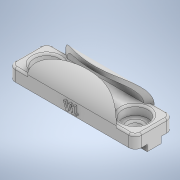
# Autodesk Inventor part: Cable Management
Saved by Autodesk Inventor 2020 (Build 240168000, 168)
## iProperties
Created: 2020-02-15
Part Number: Cable Management
Material: Generic
Document SubType Name: Modeling
Designer: maple
Density: 1 g/cm^3
Appearance: Default
Author: maple
Autodesk Inventor part; units mm, degrees
ref_plane "YZ Plane" through (0, 0, 0) normal (1, 0, 0) x (0, 1, 0)
ref_plane "XZ Plane" through (0, 0, 0) normal (0, 1, 0) x (-1, 0, 0)
ref_plane "XY Plane" through (0, 0, 0) normal (0, 0, 1) x (1, 0, 0)
sketch "Sketch1" plane through (0, 0, 0) normal (0, 1, 0) x (-1, 0, 0)
  line L0 (0, 0) -> (-50.8, 0)
  line L1 (-50.8, 0) -> (-50.8, -15.24)
  line L2 (-50.8, -15.24) -> (0, -15.24)
  line L3 (0, -15.24) -> (0, 0)
  dimension "d0" = 50.8
  dimension "d1" = 15.24
  constraints: 8 end point, 2 parallel, 1 horizontal, 1 perpendicular
  measures "d0" distance of L2.end L1.end
  measures "d1" distance of L1.end L0.end
extrude "Extrusion1" add sketch "Sketch1" along normal blind 5.08
sketch "Sketch2" plane through (0, 0, 0) normal (0, -1, 0) x (1, 0, 0)
  line L0 (0, -15.24) -> (0, 0) projected
  line L1 (0, -7.62) -> (0, -4.826)
  line L2 (0, -7.62) -> (0, -10.414)
  line L3 (0, -4.826) -> (50.8, -4.826)
  line L4 (50.8, -4.826) -> (50.8, -10.414)
  line L5 (50.8, -10.414) -> (0, -10.414)
  line L6 (0, -10.414) -> (0, -4.826)
  dimension "d4" = 2.794
  dimension "d5" = 2.794
  constraints: 12 end point, 2 parallel, 2 point on line, 1 horizontal, 1 midpoint, 1 perpendicular
  measures "d4" distance of L1.start L1.end
  measures "d5" distance of L1.start L2.end
extrude "Extrusion2" add sketch "Sketch2" along normal blind 2.54
sketch "Sketch3" plane through (0, 5.08, 0) normal (0, 1, 0) x (1, 0, 0)
  line L0 (0, 15.24) -> (0, 0) projected
  line L1 (0, 7.62) -> (7.62, 7.62)
  line L2 (50.8, 0) -> (50.8, 15.24) projected
  line L3 (50.8, 7.62) -> (43.18, 7.62)
  dimension "d8" = 7.62
  dimension "d9" = 7.62
  constraints: 4 end point, 2 horizontal, 2 midpoint
  measures "d8" distance of L1.start L1.end
  measures "d9" distance of L3.start L3.end
hole "Hole1" at (7.62, 5.08, -7.62) at (43.18, 5.08, -7.62) direction (0, -1, 0) diameter 5.08 end through all counterbore diameter 10.16 counterbore depth 3.81
sketch "Sketch4" plane through (0, 5.08, 0) normal (0, 1, 0) x (1, 0, 0)
  circle A0 centre (7.62, 7.62) radius 5.08 projected
  line L0 (7.62, 7.62) -> (7.62, 0)
  circle A1 centre (43.18, 7.62) radius 5.08 projected
  line L1 (43.18, 7.62) -> (43.18, 15.24)
  line L2 (50.8, 15.24) -> (0, 15.24) projected
  line L3 (7.62, 0) -> (43.18, 0)
  line L4 (43.18, 0) -> (43.18, 15.24)
  line L5 (43.18, 15.24) -> (7.62, 15.24)
  line L6 (7.62, 15.24) -> (7.62, 0)
  line L7 (7.62, 7.62) -> (43.18, 7.62)
  line L8 (25.4, 7.62) -> (25.4, 6.35)
  line L9 (25.4, 6.35) -> (25.4, 8.89)
  arc A2 (7.62, 15.24) -> (43.18, 15.24) centre (25.4, 36.957) ccw
  arc A3 (43.18, 0) -> (7.62, 0) centre (25.4, -21.717) ccw
  point P0 (0, 0)
  dimension "d17" = 1.27
  dimension "d18" = 2.54
  constraints: 18 end point, 6 point on circle, 3 vertical, 2 centre point, 2 parallel, 2 perpendicular, 2 point on line, 1 horizontal, 1 midpoint
  measures "d17" distance of L8.start L8.end
  measures "d18" distance of L8.end L9.end
extrude "Extrusion3" add sketch "Sketch4" along normal blind 7.62 contours L2 A2 | A3 L3
sketch "Sketch5" plane through (50.8, 0, -15.24) normal (1, 0, 0) x (0, 0, -1)
  line L0 (-1.3559, 12.7) -> (-6.35, 12.7) projected
  line L1 (-8.89, 12.7) -> (-13.8841, 12.7) projected
  line L2 (-6.35, 12.7) -> (-8.89, 12.7)
  line L3 (-7.62, 12.7) -> (-7.62, 10.922)
  line L4 (0, 5.08) -> (0, 12.7) projected
  line L5 (0, 5.08) -> (-1.778, 5.08)
  line L6 (-6.35, 5.08) -> (0, 5.08) projected
  line L7 (-15.24, 5.08) -> (-15.24, 12.7) projected
  line L8 (-15.24, 5.08) -> (-13.462, 5.08)
  line L9 (-15.24, 5.08) -> (-8.89, 5.08) projected
  arc A0 (-1.778, 5.08) -> (-13.462, 5.08) centre (-7.62, 5.08) ccw
  arc A1 (0, 5.08) -> (-15.24, 5.08) centre (-7.62, 5.08) ccw
  line L10 (0, 0) -> (0, 5.08) projected
  line L11 (0, 5.08) -> (-15.24, 5.08)
  line L12 (-15.24, 5.08) -> (-15.24, 12.7)
  line L13 (-15.24, 12.7) -> (0, 12.7)
  line L14 (0, 12.7) -> (0, 5.08)
  point P0 (-15.24, 0)
  point P1 (0, 8.3228)
  point P2 (-15.24, 8.3228)
  dimension "d22" = 1.778
  dimension "d23" = 1.778
  dimension "d24" = 1.778
  constraints: 16 end point, 6 point on circle, 2 centre point, 2 horizontal, 2 parallel, 2 point on line, 2 tangent, 1 midpoint, 1 perpendicular, 1 vertical
  measures "d22" distance of L3.start L3.end
  measures "d23" distance of L4.start L5.end
  measures "d24" distance of L7.start L8.end
extrude "Extrusion4" cut sketch "Sketch5" against normal blind 50.8 contours L13 L4 A1 L2 L0 | A1 L7 L13 L1 L2 | A0 L6 L11 L9
fillet "Fillet2" radius 2.54 4 edges at (0, 2.54, 0) (0, 2.54, -15.24) (50.8, 2.54, 0) (50.8, 2.54, -15.24)
sketch "Sketch6" plane through (7.62, 5.08, 0) normal (0, 0, 1) x (1, 0, 0)
  line L0 (0, 0) -> (35.56, 0) projected
  line L1 (17.78, 0) -> (17.78, -5.08)
  line L2 (43.18, -5.08) -> (-7.62, -5.08) projected
  line L3 (15.4127, -0.9362) -> (20.2021, -0.9362) construction
  line L4 (20.2021, -0.9362) -> (20.2021, -3.9941) construction
  line L5 (20.2021, -3.9941) -> (15.4127, -3.9941) construction
  line L6 (15.4127, -3.9941) -> (15.4127, -0.9362) construction
  line L7 (17.9186, -0.9448) -> (16.8713, -3.9928)
  line L8 (16.8713, -3.9928) -> (16.0735, -3.9928)
  line L9 (16.0735, -3.9928) -> (15.0262, -0.9448)
  line L10 (15.0262, -0.9448) -> (15.819, -0.9448)
  line L11 (15.819, -0.9448) -> (16.4835, -3.0122)
  line L12 (16.4835, -3.0122) -> (17.1454, -0.9448)
  line L13 (17.1454, -0.9448) -> (17.9186, -0.9448)
  line L14 (20.2997, -3.9928) -> (18.2866, -3.9928)
  line L15 (18.2866, -3.9928) -> (18.2866, -3.4618)
  line L16 (18.2866, -3.4618) -> (18.9288, -3.4618)
  line L17 (18.9288, -3.4618) -> (18.9288, -1.8488)
  line L18 (18.9288, -1.8488) -> (18.2866, -1.8488)
  line L19 (18.2866, -1.8488) -> (18.2866, -1.3524)
  spline S0 degree 2 poles (18.2866, -1.3524) (18.4274, -1.3524) (18.7065, -1.3153) (18.7905, -1.2758) knots 0 0 0 1 2 2 2
  spline S1 degree 2 poles (18.7905, -1.2758) (18.8868, -1.2264) (18.9955, -1.0609) (19.0054, -0.9374) knots 0 0 0 1 2 2 2
  line L20 (19.0054, -0.9374) -> (19.6723, -0.9374)
  line L21 (19.6723, -0.9374) -> (19.6723, -3.4618)
  line L22 (19.6723, -3.4618) -> (20.2997, -3.4618)
  line L23 (20.2997, -3.4618) -> (20.2997, -3.9928)
  point P0 (17.78, -2.54)
  constraints: 3 midpoint, 2 end point, 2 other
emboss "Emboss1" sketch "Sketch6" operation add depth 0.762 direction (0, 0, -1)
fillet "Fillet3" radius 0.762 14 edges at (50.0561, 5.08, -0.7439) (50.8, 5.08, -7.62) (50.0561, 5.08, -14.4961) (45.72, 5.08, -15.24) (45.72, 5.08, 0) (0.7439, 5.08, -0.7439) (0, 5.08, -7.62) (0.7439, 5.08, -14.4961) (5.08, 5.08, -15.24) (5.08, 5.08, 0) (43.18, 5.08, -12.7) (7.62, 5.08, -12.7) (7.62, 1.27, -10.16) (43.18, 1.27, -10.16)
body "Solid1"
